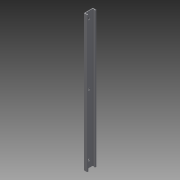
# Autodesk Inventor part: SAR330-30_b
Saved by Autodesk Inventor 2014 SP2 (Build 180246200, 246)
## iProperties
Created: 2019-04-19
Part Number: SAR330-30_b
Material: Generic
Catalog Web Link: www.cadenas.de
Description: SAR3_body-Slide Rails - Aluminum Alloy - Three - Step Slide Rails
Vendor: MISUMI
Document SubType Name: Modeling
Designer: psadmin
Manufacturer: MISUMI
Mass: 16.0078 g
Surface Area: 203.079 cm^2
Volume: 16.0078 cm^3
Density: 1 g/cm^3
Appearance: PSOLRGB-192-192-192
Category: PARTsolutions
Company: MISUMI
Title: SAR330-30
Author: Cadenas PARTsolutions
Comments: Slide Rails - Aluminum Alloy - Three - Step Slide Rails
PSOL_IDENT_0: {$CADENAS_DATA\23d-libs\misumi\metric\07_slide_rails\sar3_series\sar3_body.prj},167 {VTYP=3D},{NB=SA
PSOL_IDENT_1: R330-30_b},{LINA=SAR330-30},{NN=SAR3_body},{DATE=30.03.2018 01:39:43},{GEOMDATE=01.03.2017 01:13:00}
PSOL_IDENT_2: ,{VERSION=},{LINEID=10},{WBVAR=NO},{WBNUMERIC=NO}  {NB=SAR330-30_b},{LINA=SAR330-30},{KT=DUMMY},{PN=
PSOL_IDENT_3: SAR330-30},{TYPE=SAR330},{MAT1=Aluminum Alloy},{ST1=Clear Anodizing},{MAT2=Aluminum Alloy},{ST2=Clea
PSOL_IDENT_4: r Anodizing},{MAT3=Steel},{NO=30},{RL=300},{TD=345},{A=135},{B=270},{C=135},{D=270},{RLO=147},{BA=25
PSOL_IDENT_5: },{PPATH=sar3_series\\sar3_templ.prj}
NN: SAR3_body
NT: Slide Rails - Aluminum Alloy - Three - Step Slide Rails
NB: SAR330-30_b
NBSYN: $PN._b
LINA: SAR330-30
PN: SAR330-30
TYPE: SAR330
MAT1: Aluminum Alloy
ST1: Clear Anodizing
MAT2: Aluminum Alloy
ST2: Clear Anodizing
MAT3: Steel
NO: 30
RL: 300
TD: 345
RLO: 147
SUPPLIER: MISUMI
ARTICLENO: SAR330-30_b
BOMINFO: SAR330-30
CREATOR: CADENAS GmbH
Autodesk Inventor part; units mm, degrees
ref_plane "YZ Plane" through (0, 0, 0) normal (1, 0, 0) x (0, 1, 0)
ref_plane "XZ Plane" through (0, 0, 0) normal (0, 1, 0) x (-1, 0, 0)
ref_plane "XY Plane" through (0, 0, 0) normal (0, 0, 1) x (1, 0, 0)
sketch "Sketch_1" plane through (0, 0, 0) normal (0, 0, 1) x (1, 0, 0)
  line L0 (-7.4, 0.7071) -> (-6.6929, 0)
  line L1 (-6.6929, 0) -> (0, 0)
  line L2 (0, 0) -> (0, 2.5)
  line L3 (0, 2.5) -> (-2.3335, 2.5)
  arc A0 (-5.2665, 2.5) -> (-2.3335, 2.5) centre (-3.8, 3.2) ccw
  line L4 (-5.2665, 2.5) -> (-6, 2.5)
  line L5 (-6, 2.5) -> (-6, 17.5)
  line L6 (-6, 17.5) -> (-5.2665, 17.5)
  arc A1 (-2.3335, 17.5) -> (-5.2665, 17.5) centre (-3.8, 16.8) ccw
  line L7 (-2.3335, 17.5) -> (0, 17.5)
  line L8 (0, 17.5) -> (0, 20)
  line L9 (0, 20) -> (-6.6929, 20)
  line L10 (-6.6929, 20) -> (-7.4, 19.2929)
  line L11 (-7.4, 19.2929) -> (-7.4, 0.7071)
  constraints: 24 end point, 4 point on circle, 2 centre point
extrude "Extrusion1" add sketch "Sketch_1" along normal blind 300
sketch "Sketch_2" plane through (0, 0, 15) normal (0, 0, 1) x (1, 0, 0)
  line L0 (-6, 10) -> (-7.4, 10)
  line L1 (-7.4, 10) -> (-7.4, 11.65)
  line L2 (-7.4, 11.65) -> (-6, 13.05)
  line L3 (-6, 13.05) -> (-6, 10)
  line L4 (-6, 10) -> (-7.4, 10)
  constraints: 10 end point
revolve "Revolution1" cut sketch "Sketch_2" angle 360 about axis through (-6, 10, 15) along (1, 0, 0)
pattern_linear "Rectangular Pattern1" count 3 spacing 135 along (0, 0, 1) of "Revolution1"
ref_plane "to_ball_XY" through (-3.8, 3.25, 111) normal (0, 0, 1) x (1, 0, 0)
ref_plane "to_ball_YZ" through (-3.8, 3.25, 111) normal (1, 0, 0) x (0, 1, 0)
ref_plane "to_ball_ZX" through (-3.8, 3.25, 111) normal (0, 1, 0) x (0, 0, 1)
ref_plane "to_ball1_XY" through (-3.8, 16.75, 111) normal (0, 0, 1) x (1, 0, 0)
ref_plane "to_ball1_YZ" through (-3.8, 16.75, 111) normal (1, 0, 0) x (0, 1, 0)
ref_plane "to_ball1_ZX" through (-3.8, 16.75, 111) normal (0, 1, 0) x (0, 0, 1)
ref_plane "to_rail_XY" through (0.6, 10, 150) normal (0, 0, 1) x (1, 0, 0)
ref_plane "to_rail_YZ" through (0.6, 10, 150) normal (1, 0, 0) x (0, 1, 0)
ref_plane "to_rail_ZX" through (0.6, 10, 150) normal (0, 1, 0) x (0, 0, 1)
body "Solid1"
